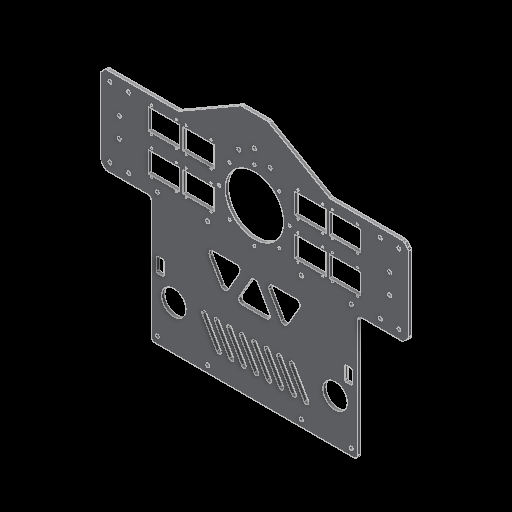
# Autodesk Inventor part: Root
Saved by Autodesk Inventor 2025.2 (Build 292293000, 293)
## iProperties
Created: 2020-05-07
Part Number: Root
Material: Generic
Document SubType Name: Sheet Metal
Designer: valer
Density: 1 g/cm^3
Sheet Metal Rule: Default
Appearance: Default
Author: valer
Autodesk Inventor part; units mm, degrees
ref_plane "YZ Plane" through (0, 0, 0) normal (1, 0, 0) x (0, 1, 0)
ref_plane "XZ Plane" through (0, 0, 0) normal (0, 1, 0) x (-1, 0, 0)
ref_plane "XY Plane" through (0, 0, 0) normal (0, 0, 1) x (1, 0, 0)
sketch "Base" plane through (0, 0, 0) normal (0, 0, 1) x (1, 0, 0)
  circle A0 centre (-56.25, 0) radius 2.75 construction
  circle A1 centre (0, -56.25) radius 2.75 construction
  circle A2 centre (0, 56.25) radius 2.75 construction
  circle A3 centre (39.7748, -39.7748) radius 2.75 construction
  circle A4 centre (-39.7748, 39.7748) radius 2.75 construction
  circle A5 centre (-39.7748, -39.7748) radius 2.75 construction
  circle A6 centre (39.7748, 39.7748) radius 2.75 construction
  circle A7 centre (56.25, 0) radius 2.75 construction
  circle A8 centre (0, 0) radius 45 construction
  circle A9 centre (0, 0) radius 61
  line L0 (0, -352) -> (0, 222) construction
  line L1 (-344.741, 0) -> (344.741, 0) construction
  circle A10 centre (0, 0) radius 46.5
  circle A11 centre (-56.25, 0) radius 2.25
  circle A12 centre (-39.7748, -39.7748) radius 2.25
  circle A13 centre (0, -56.25) radius 2.25
  circle A14 centre (39.7748, -39.7748) radius 2.25
  circle A15 centre (56.25, 0) radius 2.25
  circle A16 centre (39.7748, 39.7748) radius 2.25
  circle A17 centre (0, 56.25) radius 2.25
  circle A18 centre (-39.7748, 39.7748) radius 2.25
  line L2 (-121.2436, 70) -> (0, 140)
  line L3 (0, 140) -> (121.2436, 70)
  line L4 (121.2436, 70) -> (121.2436, -70)
  line L5 (121.2436, -70) -> (0, -140)
  line L6 (0, -140) -> (-121.2436, -70)
  line L7 (-121.2436, -70) -> (-121.2436, 70)
  line L8 (121.2436, 70) -> (246.2436, 70)
  line L9 (246.2436, 70) -> (246.2436, -70)
  line L10 (246.2436, -70) -> (121.2436, -70)
  line L11 (-121.2436, 70) -> (-246.2436, 70)
  line L12 (-246.2436, 70) -> (-246.2436, -70)
  line L13 (-246.2436, -70) -> (-121.2436, -70)
  line L14 (165, -70) -> (165, -270)
  line L15 (165, -270) -> (0, -270)
  line L16 (-165, -70) -> (-165, -270)
  line L17 (-165, -270) -> (0, -270)
  point P0 (0, 0)
  dimension "d91" = 1.5
  dimension "d92" = 4.5
  dimension "d164" = 125
  dimension "d165" = 140
  dimension "d173" = 165
  dimension "d174" = 200
  measures "d91" radial gap between concentric circles of A10 A8
  measures "d92" diameter of A11
  measures "d164" distance of L3.end L8.end
  measures "d165" distance of L8.end L9.end
  measures "d173" distance of L14.end L15.end
  measures "d174" distance between parallel lines of L10 L15
extrude "Plate1" add sketch "Base" against normal blind 5 contours A9 | L2 L3 L4 L5 L6 L7 | L7 L13 L12 L11 | L6 L5 L10 L14 L15 L17 L16 L13 | L8 L9 L10 L4
sketch "LegMountHoles" plane through (0, 0, -5) normal (0, 0, -1) x (-1, 0, 0)
  line L0 (-216.2436, 44.9096) -> (-216.2436, -35.0904) construction
  line L1 (-201.2436, 56) -> (-231.2436, 56) construction
  circle A0 centre (-201.2436, 56) radius 3
  circle A1 centre (-231.2436, 56) radius 3
  circle A2 centre (-216.2436, 16) radius 3
  line L2 (344.741, 0) -> (-344.741, 0) construction
  line L3 (0, -352) -> (0, 222) construction
  circle A3 centre (201.2436, 56) radius 3
  circle A4 centre (231.2436, 56) radius 3
  circle A5 centre (216.2436, 16) radius 3
  circle A6 centre (-201.2436, -56) radius 3
  circle A7 centre (-231.2436, -56) radius 3
  circle A8 centre (-216.2436, -16) radius 3
  circle A9 centre (201.2436, -56) radius 3
  circle A10 centre (231.2436, -56) radius 3
  circle A11 centre (216.2436, -16) radius 3
  line L4 (-246.2436, -70) -> (-246.2436, 70) projected
  point P0 (0, 0)
  point P1 (-216.2436, 56)
  dimension "d93" = 6
  dimension "d94" = 30
  dimension "d95" = 40
  dimension "d161" = 16
  dimension "d166" = 30
  constraints: 12 centre point, 9 symmetric about line, 4 end point, 2 coincident, 2 equal radius, 2 point on line, 1 horizontal, 1 midpoint, 1 perpendicular, 9 other
  measures "d93" diameter of A0
  measures "d94" distance of L1.start L1.end
  measures "d95" distance from line of L1 A2.centre
  measures "d161" distance from line of L2 A2.centre
  measures "d166" distance between parallel lines of L4 L0
extrude "LegMountHolesFeature" cut sketch "LegMountHoles" against normal blind 5
chamfer "FrontChamferFeature" distance 25 angle 45 1 edges at (0, 140, -2.5)
chamfer "SideChamfersFeature" distance 8 angle 45 4 edges at (246.2436, 70, -2.5) (246.2436, -70, -2.5) (-246.2436, 70, -2.5) (-246.2436, -70, -2.5)
fillet "FilletsFeature" radius 6 16 edges at (165, -270, -2.5) (-165, -270, -2.5) (-238.2436, -70, -2.5) (-246.2436, -62, -2.5) (-165, -70, -2.5) (165, -70, -2.5) (238.2436, -70, -2.5) (246.2436, -62, -2.5) (246.2436, 62, -2.5) (238.2436, 70, -2.5) (121.2436, 70, -2.5) (21.6506, 127.5, -2.5) (-21.6506, 127.5, -2.5) (-121.2436, 70, -2.5) (-238.2436, 70, -2.5) (-246.2436, 62, -2.5)
sketch "BatteryContactHoles" plane through (0, 0, -5) normal (0, 0, -1) x (-1, 0, 0)
  circle A0 centre (-129.1, -199.15) radius 18.4 construction
  circle A1 centre (129.1, -199.15) radius 18.4 construction
  circle A2 centre (129.1, -199.15) radius 19.4
  circle A3 centre (-129.1, -199.15) radius 19.4
  point P0 (0, 0)
  dimension "d199" = 1
  constraints: 2 centre point, 2 coincident, 1 equal radius
  measures "d199" radial gap between concentric circles of A2 A1
extrude "BatteryContactHolesFeature" cut sketch "BatteryContactHoles" against normal blind 5
sketch "BatteryMountHoles" plane through (0, 0, -5) normal (0, 0, -1) x (-1, 0, 0)
  circle A0 centre (-155, -259) radius 3 projected
  circle A1 centre (-75, -259) radius 3 projected
  circle A2 centre (75, -259) radius 3 projected
  circle A3 centre (155, -259) radius 3 projected
  circle A4 centre (-155, -59.5) radius 3 projected
  circle A5 centre (-75, -59.5) radius 3 projected
  circle A6 centre (75, -59.5) radius 3 projected
  circle A7 centre (155, -59.5) radius 3 projected
  point P0 (0, 0)
extrude "BatteryMountHolesFeature" cut sketch "BatteryMountHoles" against normal blind 5
sketch "BatteryStrapHoles" plane through (0, 0, -5) normal (0, 0, -1) x (-1, 0, 0)
  line L0 (-156.75, -148) -> (-144.75, -148)
  line L1 (-144.75, -148) -> (-144.75, -171.5)
  line L2 (-144.75, -171.5) -> (-156.75, -171.5)
  line L3 (-156.75, -171.5) -> (-156.75, -148)
  line L4 (0, -349.5) -> (0, 207) construction
  line L5 (-156.75, -148) -> (-152.25, -148) projected
  line L6 (-152.25, -171.5) -> (-156.75, -171.5) projected
  line L7 (156.75, -148) -> (144.75, -148)
  line L8 (144.75, -148) -> (144.75, -171.5)
  line L9 (144.75, -171.5) -> (156.75, -171.5)
  line L10 (156.75, -171.5) -> (156.75, -148)
  point P0 (0, 0)
  dimension "d204" = 12
  constraints: 16 end point, 4 symmetric about line, 2 parallel, 1 horizontal, 1 perpendicular
  measures "d204" distance of L0.start L0.end
extrude "BatteryStrapHolesFeature" cut sketch "BatteryStrapHoles" against normal blind 5
fillet "BatteryStrapHoleFilletsFeature" radius 2 8 edges at (156.75, -148, -2.5) (144.75, -148, -2.5) (156.75, -171.5, -2.5) (144.75, -171.5, -2.5) (-144.75, -148, -2.5) (-156.75, -148, -2.5) (-156.75, -171.5, -2.5) (-144.75, -171.5, -2.5)
sketch "BaseCuts" plane through (0, 0, -5) normal (0, 0, -1) x (-1, 0, 0)
  line L0 (-77.3649, -96.25) -> (-47.9201, -147.25)
  line L1 (-47.9201, -147.25) -> (-18.4752, -96.25)
  line L2 (-18.4752, -96.25) -> (-77.3649, -96.25)
  line L3 (-66.3953, -147.25) -> (-95.8401, -96.25)
  line L4 (-95.8401, -96.25) -> (-125.285, -147.25)
  line L5 (-125.285, -147.25) -> (-66.3953, -147.25)
  line L6 (0, -349.5) -> (0, 207) construction
  line L7 (77.3649, -96.25) -> (47.9201, -147.25)
  line L8 (47.9201, -147.25) -> (18.4752, -96.25)
  line L9 (18.4752, -96.25) -> (77.3649, -96.25)
  line L10 (66.3953, -147.25) -> (95.8401, -96.25)
  line L11 (95.8401, -96.25) -> (125.285, -147.25)
  line L12 (125.285, -147.25) -> (66.3953, -147.25)
  line L13 (359.0244, -147.25) -> (-330.4576, -147.25) construction
  line L14 (-125.285, -163.25) -> (-66.3953, -163.25)
  line L15 (-66.3953, -163.25) -> (-95.8401, -214.25)
  line L16 (-95.8401, -214.25) -> (-125.285, -163.25)
  line L17 (-66.3953, -147.25) -> (-66.3953, -163.25) construction
  line L18 (125.285, -163.25) -> (66.3953, -163.25)
  line L19 (66.3953, -163.25) -> (95.8401, -214.25)
  line L20 (95.8401, -214.25) -> (125.285, -163.25)
  line L21 (18.4752, -96.25) -> (-18.4752, -96.25) construction
  line L22 (0, -96.25) -> (29.4449, -147.25)
  line L23 (0, -96.25) -> (-29.4449, -147.25)
  line L24 (-29.4449, -147.25) -> (29.4449, -147.25)
  circle A0 centre (0, -56.25) radius 2.25 projected
  point P0 (0, 0)
  dimension "d218" = 60
  dimension "d219" = 60
  dimension "d242" = 51
  dimension "d244" = 16
  dimension "d246" = 16
  dimension "d247" = 60
  dimension "d248" = 60
  dimension "d255" = 16
  dimension "d256" = 40
  constraints: 46 end point, 9 symmetric about line, 7 horizontal, 3 equal length, 3 parallel, 1 midpoint, 1 vertical, 6 other
  measures "d218" angle of L5 L3
  measures "d219" angle of L4 L5
  measures "d242" distance from line of L5 L3.end
  measures "d244" distance between parallel lines of L3 L0
  measures "d246" distance between parallel lines of L14 L5
  measures "d247" angle of L15 L14
  measures "d248" angle of L16 L14
  measures "d255" distance between parallel lines of L22 L8
  measures "d256" distance from line of L21 A0.centre
extrude "BaseCutsFeature" cut sketch "BaseCuts" against normal blind 5 contours L2 L1 L0 | L7 L8 L9 | L22 L24 L23
fillet "BaseCutFilletsFeature" radius 6 9 edges at (18.4752, -96.25, -2.5) (77.3649, -96.25, -2.5) (47.9201, -147.25, -2.5) (-77.3649, -96.25, -2.5) (-18.4752, -96.25, -2.5) (-47.9201, -147.25, -2.5) (0, -96.25, -2.5) (-29.4449, -147.25, -2.5) (29.4449, -147.25, -2.5)
sketch "BackVents" plane through (0, 0, -5) normal (0, 0, -1) x (-1, 0, 0)
  line L0 (-83, -230) -> (-59.906, -190) construction
  line L1 (-86.4641, -228) -> (-63.3701, -188)
  line L2 (-56.4419, -192) -> (-79.5359, -232)
  arc A0 (-86.4641, -228) -> (-79.5359, -232) centre (-83, -230) ccw
  arc A1 (-56.4419, -192) -> (-63.3701, -188) centre (-59.906, -190) ccw
  line L3 (344.741, 0) -> (-344.741, 0) construction
  line L4 (0, -349.5) -> (0, 207) construction
  line L5 (159, -270) -> (-159, -270) projected
  line L6 (-83, -230) -> (165, -230) construction
  line L7 (-59.906, -190) -> (165, -190) construction
  line L8 (-165, -264) -> (-165, -76) projected
  line L9 (165, -76) -> (165, -264) projected
  arc A2 (-36.4419, -192) -> (-43.3701, -188) centre (-39.906, -190) ccw
  line L10 (-66.4641, -228) -> (-43.3701, -188)
  line L11 (-36.4419, -192) -> (-59.5359, -232)
  arc A3 (-66.4641, -228) -> (-59.5359, -232) centre (-63, -230) ccw
  arc A4 (-16.4419, -192) -> (-23.3701, -188) centre (-19.906, -190) ccw
  line L12 (-46.4641, -228) -> (-23.3701, -188)
  line L13 (-16.4419, -192) -> (-39.5359, -232)
  arc A5 (-46.4641, -228) -> (-39.5359, -232) centre (-43, -230) ccw
  arc A6 (3.5581, -192) -> (-3.3701, -188) centre (0.094, -190) ccw
  line L14 (-26.4641, -228) -> (-3.3701, -188)
  line L15 (3.5581, -192) -> (-19.5359, -232)
  arc A7 (-26.4641, -228) -> (-19.5359, -232) centre (-23, -230) ccw
  arc A8 (23.5581, -192) -> (16.6299, -188) centre (20.094, -190) ccw
  line L16 (-6.4641, -228) -> (16.6299, -188)
  line L17 (23.5581, -192) -> (0.4641, -232)
  arc A9 (-6.4641, -228) -> (0.4641, -232) centre (-3, -230) ccw
  arc A10 (43.5581, -192) -> (36.6299, -188) centre (40.094, -190) ccw
  line L18 (13.5359, -228) -> (36.6299, -188)
  line L19 (43.5581, -192) -> (20.4641, -232)
  arc A11 (13.5359, -228) -> (20.4641, -232) centre (17, -230) ccw
  arc A12 (63.5581, -192) -> (56.6299, -188) centre (60.094, -190) ccw
  line L20 (33.5359, -228) -> (56.6299, -188)
  line L21 (63.5581, -192) -> (40.4641, -232)
  arc A13 (33.5359, -228) -> (40.4641, -232) centre (37, -230) ccw
  arc A14 (83.5581, -192) -> (76.6299, -188) centre (80.094, -190) ccw
  line L22 (53.5359, -228) -> (76.6299, -188)
  line L23 (83.5581, -192) -> (60.4641, -232)
  arc A15 (53.5359, -228) -> (60.4641, -232) centre (57, -230) ccw
  point P0 (0, 0)
  point P1 (-71.453, -210)
  dimension "d223" = 4
  dimension "d224" = 40
  dimension "d225" = 80
  dimension "d226" = 60
  dimension "d227" = 82
  dimension "d230" = 20
  constraints: 40 end point, 32 point on circle, 16 centre point, 4 tangent, 3 horizontal, 2 point on line, 1 midpoint, 1 parallel, 70 other
  measures "d223" radius of A1
  measures "d224" distance from line of L5 L0.start
  measures "d225" distance from line of L5 L0.end
  measures "d226" angle of L0 L6
  measures "d227" distance from line of L8 L0.start
  measures "d230" distance of L0.end A2.centre
extrude "VentsFeature" cut sketch "BackVents" against normal blind 5
sketch "LaserMountHoles" plane through (0, 0, -5) normal (0, 0, -1) x (-1, 0, 0)
  circle A0 centre (25, 65) radius 3 projected
  circle A1 centre (0, 79) radius 3 projected
  circle A2 centre (-25, 65) radius 3 projected
  point P0 (0, 0)
extrude "LaserMountHolesFeature" cut sketch "LaserMountHoles" against normal blind 5
sketch "MotorDriverMountHoles" plane through (0, 0, -5) normal (0, 0, -1) x (-1, 0, 0)
  circle A0 centre (-164.6136, 16.15) radius 1.65 projected
  circle A1 centre (-164.6136, 56.35) radius 1.65 projected
  circle A2 centre (-125.2136, 16.15) radius 1.65 projected
  circle A3 centre (-125.2136, 56.35) radius 1.65 projected
  circle A4 centre (-125.2136, -3.15) radius 1.65 projected
  circle A5 centre (-164.6136, -3.15) radius 1.65 projected
  circle A6 centre (-164.6136, -43.35) radius 1.65 projected
  circle A7 centre (-125.2136, -43.35) radius 1.65 projected
  circle A8 centre (-109.1136, -43.35) radius 1.65 projected
  circle A9 centre (-109.1136, -3.15) radius 1.65 projected
  circle A10 centre (-69.7136, -3.15) radius 1.65 projected
  circle A11 centre (-69.7136, -43.35) radius 1.65 projected
  circle A12 centre (-109.1136, 16.15) radius 1.65 projected
  circle A13 centre (-109.1136, 56.35) radius 1.65 projected
  circle A14 centre (-69.7136, 56.35) radius 1.65 projected
  circle A15 centre (-69.7136, 16.15) radius 1.65 projected
  line L0 (0, -349.5) -> (0, 207) construction
  circle A16 centre (164.6136, 16.15) radius 1.65
  circle A17 centre (164.6136, 56.35) radius 1.65
  circle A18 centre (125.2136, 16.15) radius 1.65
  circle A19 centre (125.2136, 56.35) radius 1.65
  circle A20 centre (125.2136, -3.15) radius 1.65
  circle A21 centre (164.6136, -3.15) radius 1.65
  circle A22 centre (164.6136, -43.35) radius 1.65
  circle A23 centre (125.2136, -43.35) radius 1.65
  circle A24 centre (109.1136, -43.35) radius 1.65
  circle A25 centre (109.1136, -3.15) radius 1.65
  circle A26 centre (69.7136, -3.15) radius 1.65
  circle A27 centre (69.7136, -43.35) radius 1.65
  circle A28 centre (109.1136, 16.15) radius 1.65
  circle A29 centre (109.1136, 56.35) radius 1.65
  circle A30 centre (69.7136, 56.35) radius 1.65
  circle A31 centre (69.7136, 16.15) radius 1.65
  line L1 (-120.1636, 51.5) -> (-169.6636, 51.5) construction
  line L2 (-169.6636, 19) -> (-120.1636, 19) construction
  line L3 (-169.6636, 57.1) -> (-169.6636, 15.2) construction
  line L4 (-120.1636, 29.86) -> (-120.1636, 57.1) construction
  line L5 (-169.9136, 51.75) -> (-119.9136, 51.75)
  line L6 (-119.9136, 51.75) -> (-119.9136, 18.75)
  line L7 (-119.9136, 18.75) -> (-169.9136, 18.75)
  line L8 (-169.9136, 18.75) -> (-169.9136, 51.75)
  line L9 (-169.9136, 51.75) -> (-119.9136, 18.75) construction
  line L10 (-114.4136, 51.75) -> (-64.4136, 51.75)
  line L11 (-64.4136, 51.75) -> (-64.4136, 18.75)
  line L12 (-64.4136, 18.75) -> (-114.4136, 18.75)
  line L13 (-114.4136, 18.75) -> (-114.4136, 51.75)
  line L14 (-169.9136, -7.75) -> (-119.9136, -7.75)
  line L15 (-119.9136, -7.75) -> (-119.9136, -40.75)
  line L16 (-119.9136, -40.75) -> (-169.9136, -40.75)
  line L17 (-169.9136, -40.75) -> (-169.9136, -7.75)
  line L18 (-114.4136, -7.75) -> (-64.4136, -7.75)
  line L19 (-64.4136, -7.75) -> (-64.4136, -40.75)
  line L20 (-64.4136, -40.75) -> (-114.4136, -40.75)
  line L21 (-114.4136, -40.75) -> (-114.4136, -7.75)
  line L22 (169.9136, 51.75) -> (119.9136, 51.75)
  line L23 (119.9136, 51.75) -> (119.9136, 18.75)
  line L24 (119.9136, 18.75) -> (169.9136, 18.75)
  line L25 (169.9136, 18.75) -> (169.9136, 51.75)
  line L26 (114.4136, 51.75) -> (64.4136, 51.75)
  line L27 (64.4136, 51.75) -> (64.4136, 18.75)
  line L28 (64.4136, 18.75) -> (114.4136, 18.75)
  line L29 (114.4136, 18.75) -> (114.4136, 51.75)
  line L30 (169.9136, -7.75) -> (119.9136, -7.75)
  line L31 (119.9136, -7.75) -> (119.9136, -40.75)
  line L32 (119.9136, -40.75) -> (169.9136, -40.75)
  line L33 (169.9136, -40.75) -> (169.9136, -7.75)
  line L34 (114.4136, -7.75) -> (64.4136, -7.75)
  line L35 (64.4136, -7.75) -> (64.4136, -40.75)
  line L36 (64.4136, -40.75) -> (114.4136, -40.75)
  line L37 (114.4136, -40.75) -> (114.4136, -7.75)
  point P0 (0, 0)
  dimension "d200" = 5
  dimension "d259" = 0.25
  dimension "d260" = 0.25
  dimension "d261" = 0.25
  dimension "d262" = 0.25
  dimension "d263" = 50
  dimension "d264" = 33
  dimension "d265" = 2.6
  dimension "d266" = 5.3
  dimension "d267" = 5.3
  dimension "d268" = 5.3
  dimension "d269" = 5.3
  dimension "d270" = 2.6
  constraints: 66 end point, 32 symmetric about line, 16 centre point, 8 parallel, 6 equal length, 4 horizontal, 4 perpendicular, 2 point on line, 1 collinear, 16 other
  measures "d259" distance between parallel lines of L7 L2
  measures "d260" distance between parallel lines of L8 L3
  measures "d261" distance between parallel lines of L5 L1
  measures "d262" distance between parallel lines of L6 L4
  measures "d263" distance of L6.end L7.end
  measures "d264" distance of L7.end L5.start
  measures "d265" distance from line of L7 A2.centre
  measures "d266" distance from line of A2.centre L6
  measures "d267" distance from line of L11 A15.centre
  measures "d268" distance from line of A7.centre L15
  measures "d269" distance from line of L19 A11.centre
  measures "d270" distance from line of A7.centre L16
extrude "MotorDriverHolesFeature" cut sketch "MotorDriverMountHoles" against normal blind 5
equation "\"d97\" = Thickness"
equation "\"d33\" = Thickness"
equation "\"BendRadius\" = Thickness"
equation "\"BendReliefWidth\" = Thickness"
equation "\"BendReliefDepth\" = 0.5 * Thickness"
equation "\"TransitionRadius\" = BendRadius"
equation "\"JacobiRadiusSize\" = BendRadius"
equation "\"GapSize\" = Thickness"
equation "\"Thickness\" = 5"
body "Solid1"
